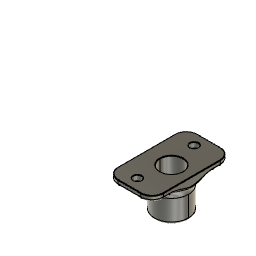
CurtainRodBracket_F3-01_004 (Side Mount) (Autodesk Fusion 360 design; units mm, degrees)
Autodesk Fusion 360 part; units mm, degrees
box "BoxPrimitive1" add length 70 width 30 height 5 placed x (0, 1, 0) y (-1, 0, 0) z (0, 0, 1) at (30, -5, 0) makes body 1
box "BoxPrimitive2" add length 30 width 30 height 25 placed x (0, 1, 0) y (-1, 0, 0) z (0, 0, 1) at (30, 15, 5) bodies 1
cylinder "CylinderPrimitive1" cut diameter 20 height -40 placed x (0, 0, -1) y (0, 1, 0) z (1, 0, 0) at (30, 30, 15) bodies 1
fillet "Fillet1" radius 14 2 edges at (15, 15, 30) (15, 45, 30) on bodies 1
fillet "Fillet2" radius 10 2 edges at (15, 15, 5) (15, 45, 5) on bodies 1
box "BoxPrimitive4" add length 20 width 30 height 7 placed x (0, 1, 0) y (1, 0, 0) z (0, 0, -1) at (0, -5, 0) bodies 1
cylinder "CylinderPrimitive3" cut diameter 7 height 21 placed x (1, 0, 0) y (0, 1, 0) z (0, 0, 1) at (15, 5, 0) bodies 1
cylinder "CylinderPrimitive4" cut diameter 20 height 34 placed x (1, 0, 0) y (0, 1, 0) z (0, 0, 1) at (15, 5, 5) bodies 1
fillet "Fillet3" radius 1.4 1 edges at (15, 15, 5) on bodies 1
fillet "Fillet4" radius 5 4 edges at (5.8399, 7.6914, 5.3692) (10.0517, 13.6899, 10.0517) (19.9483, 13.6899, 10.0517) (24.1593, 7.6637, 5.3615) on bodies 1
ref_plane "WorkPlane1" through (15, 30, 2.5) normal (0, -1, 0) x (0, 0, 1)
fillet "Fillet5" radius 10 2 edges at (30, -5, -1) (0, -5, -1) on bodies 1
fillet "Fillet6" radius 2 19 edges at (30, 60, 5) (30, 47.9289, 7.9289) (30, 45, 15.5) (30, 40.8995, 25.8995) (30, 30, 30) (30, 19.1005, 25.8995) (30, 15, 15.5) (30, 12.0711, 7.9289) (27.0711, -2.0711, 5) (15, -5, 5) (2.9289, -2.0711, 5) (0, 12.0711, 7.9289) (0, 15, 15.5) (0, 19.1005, 25.8995) (0, 30, 30) (0, 40.8995, 25.8995) (0, 45, 15.5) (0, 47.9289, 7.9289) (0, 60, 5) on bodies 1
fillet "Fillet7" radius 1 2 edges at (30, 20.6767, 18.6162) (0, 20.6767, 11.3838) on bodies 1
box "BoxPrimitive3" cut length 65 width 106 height -57 placed x (0, 0, -1) y (1, 0, 0) z (0, -1, 0) at (-44, 30, 51.5) bodies 1
fillet "Fillet9" radius 10 2 edges at (0, 15, -3.5) (30, 15, -3.5) on bodies 1
chamfer "Chamfer2" distance 0.4 angle 45 4 edges at (15, -5, -7) (30, 5, -7) (15, 15, -7) (0, 5, -7) measured on face at (6.666, 5, -7) measured on face at (30, 14.9957, 1.3615) measured on face at (6.666, 5, -7) measured on face at (0, 14.9957, 1.3615) on bodies 1
fillet "Fillet10" radius 2 3 edges at (2.9289, 12.0711, 0) (15, 15, 0) (27.0711, 12.0711, 0) on bodies 1
fillet "Fillet11" radius 3 4 edges at (0, 8.2445, -0.662) (0, 20.8166, 0) (30, 20.8166, 0) (30, 8.2445, -0.662) on bodies 1
cylinder "CylinderPrimitive5" cut diameter 7 height -50 placed x (1, 0, 0) y (0, 1, 0) z (0, 0, 1) at (15, 5, 5) bodies 1
chamfer "Chamfer3" distance 0.4 angle 45 2 edges at (11.7369, 6.2657, 5) (16.2657, 1.7369, -7) measured on face at (14.8594, -1.4915, 5) measured on face at (14.8594, 12.5582, -7) on bodies 1
box "BoxPrimitive5" add length 1 width 2 height 0.5 placed x (0, -1, 0) y (-1, 0, 0) z (0, 0, -1) at (20, -3.5, -7) separate body makes body 2
chamfer "Chamfer4" distance 0.5 angle 45 4 edges at (20, -4, -7.5) (19, -4.5, -7.5) (19, -3.5, -7.5) (18, -4, -7.5) measured on face at (18.6667, -3.8333, -7.5) measured on face at (18.6667, -3.8333, -7.5) measured on face at (18.6667, -3.8333, -7.5) measured on face at (18.6667, -3.8333, -7.5) on bodies 2
copy_body "CopyPasteBodies1" bodies 2 makes body 3
move_body "Move1" bodies 3 to x (1, 0, 0) y (0, 1, 0) z (0, 0, 1) at (9, 9, 0)
copy_body "CopyPasteBodies2" bodies 2 makes body 4
move_body "Move2" bodies 4 to x (1, 0, 0) y (0, 1, 0) z (0, 0, 1) at (-17, 9, 0)
move_body "Move3" bodies 2 to x (0, -1, 0) y (1, 0, 0) z (0, 0, 1) at (23.5, 15.5, 0)
copy_body "CopyPasteBodies3" bodies 2 makes body 5
move_body "Move4" bodies 5 to x (1, 0, 0) y (0, 1, 0) z (0, 0, 1) at (-9, 0, 0)
copy_body "CopyPasteBodies4" bodies 2 5 makes body 6 makes body 7
move_body "Move5" bodies 6 7 to x (1, 0, 0) y (0, 1, 0) z (0, 0, 1) at (0, 17, 0)
copy_body "CopyPasteBodies5" bodies 7 makes body 8
move_body "Move6" bodies 8 to x (1, 0, 0) y (0, 1, 0) z (0, 0, 1) at (25, 0, 0)
combine "Combine1" operation add target body 1 tool bodies 2 3 4 5 6 7
mirror "Mirror1" about plane through (15, 30, 2.5) normal (0, -1, 0) of bodies 1 merged
ref_plane "WorkPlane2" through (75, 30, 13) normal (1, 0, 0) x (0, 0, -1)
box "BoxPrimitive6" add length 40 width 70 height 5 placed x (0, 0, 1) y (0, -1, 0) z (1, 0, 0) at (75, 65, -7) separate body makes body 9
cylinder "CylinderPrimitive6" add diameter 30 height 30 placed x (0, 0, -1) y (0, 1, 0) z (1, 0, 0) at (80, 30, 15) bodies 9
cylinder "CylinderPrimitive7" cut diameter 20 height -47 placed x (0, 0, -1) y (0, 1, 0) z (1, 0, 0) at (110, 30, 15) bodies 9
fillet "Fillet12" radius 10 1 edges at (80, 35.4242, 28.9849) on bodies 9
fillet "Fillet13" radius 2 1 edges at (110, 24.5758, 28.9849) on bodies 9
fillet "Fillet14" radius 1 1 edges at (110, 20.6767, 18.6162) on bodies 9
fillet "Fillet15" radius 10 4 edges at (77.5, -5, 33) (77.5, -5, -7) (77.5, 65, 33) (77.5, 65, -7) on bodies 9
cylinder "CylinderPrimitive8" cut diameter 7 height -15 placed x (0, 0, -1) y (0, 1, 0) z (1, 0, 0) at (80, 5, 10) bodies 9
cylinder "CylinderPrimitive9" cut diameter 20 height 24 placed x (0, 0, -1) y (0, 1, 0) z (1, 0, 0) at (80, 5, 10) bodies 9
fillet "Fillet16" radius 1.4 1 edges at (80, 14.8058, 11.9612) on bodies 9
fillet "Fillet17" radius 4 3 edges at (80.3437, 7.9669, 19.0446) (86.7888, 14.6582, 12.5923) (80.3437, 11.2174, 2.7922) on bodies 9
fillet "Fillet18" radius 2 14 edges at (82.8586, 30, 33) (82.8586, 30, 33) (80, 51.1747, 33) (80, 8.8253, 33) (80, 62.0711, 30.0711) (80, 65, 13) (80, 62.0711, -4.0711) (80, 48.4372, -7) (80.4606, 30, -7) (80, 11.5628, -7) (80, -2.0711, -4.0711) (80, -5, 13) (80, -2.0711, 30.0711) (80, 8.8253, 33) on bodies 9
chamfer "Chamfer5" distance 0.4 angle 45 8 edges at (75, -5, 13) (75, -2.0711, -4.0711) (75, 30, -7) (75, 62.0711, -4.0711) (75, 65, 13) (75, 62.0711, 30.0711) (75, 30, 33) (75, -2.0711, 30.0711) measured on face at (75, 56.6573, 13.4176) measured on face at (76, -4.9547, 2.0494) measured on face at (75, 56.6573, 13.4176) measured on face at (76, 64.9887, 2.5242) measured on face at (75, 56.6573, 13.4176) measured on face at (76, 55.4758, 32.9887) measured on face at (75, 56.6573, 13.4176) measured on face at (76, 4.0494, 32.9547) on bodies 9
chamfer "Chamfer6" distance 0.4 angle 45 2 edges at (75, 20.6767, 11.3838) (75, 1.7369, 8.7343) measured on face at (75, 56.3907, 13.4176) measured on face at (75, 56.3907, 13.4176) on bodies 9
chamfer "Chamfer7" distance 0.4 angle 45 1 edges at (80, 1.7369, 8.7343) measured on face at (76.9333, 4.8255, 6.5044) on bodies 9
box "BoxPrimitive7" cut length 79.8249 width 114.6289 height -125 placed x (0, 0, -1) y (1, 0, 0) z (0, -1, 0) at (47.2286, 30, 46.964) bodies 9
move_body "Move8" bodies 8 to x (0, 0, -1) y (0, 1, 0) z (1, 0, 0) at (82, -17, 45.5)
copy_body "CopyPasteBodies6" bodies 8 makes body 10
move_body "Move9" bodies 10 to x (1, 0, 0) y (0, 1, 0) z (0, 0, 1) at (0, 22, 5)
copy_body "CopyPasteBodies7" bodies 8 makes body 11
move_body "Move10" bodies 11 to x (1, 0, 0) y (0, 0, 1) z (0, -1, 0) at (0, 15, -1)
copy_body "CopyPasteBodies8" bodies 11 makes body 12
move_body "Move11" bodies 12 to x (1, 0, 0) y (0, 1, 0) z (0, 0, 1) at (0, 0, 35)
copy_body "CopyPasteBodies9" bodies 8 makes body 13
move_body "Move12" bodies 13 to x (1, 0, 0) y (0, 1, 0) z (0, 0, 1) at (0, 0, 11)
move_body "Move13" bodies 8 to x (1, 0, 0) y (0, 1, 0) z (0, 0, 1) at (0, 0, -5)
combine "Combine2" operation add target body 13 tool bodies 12 11 10 9 8
mirror "Mirror2" about plane through (15, 30, 2.5) normal (0, -1, 0) of bodies 13 merged
sketch "Sketch23" plane through (80, 0, 0) normal (1, 0, 0) x (0, 1, 0)
  line L0 (45, -5) -> (55, -5)
  arc A0 (55, -5) -> (63, 3) centre (55, 3) ccw
  line L1 (63, 3) -> (63, 23)
  arc A1 (63, 23) -> (55, 31) centre (55, 23) ccw
  line L2 (55, 31) -> (49.2094, 31)
  arc A2 (54.74, 18.5961) -> (49.2094, 31) centre (30, 15) ccw
  arc A3 (54.74, 18.5961) -> (51.4538, 2.1652) centre (55, 10) ccw
  arc A4 (45, -5) -> (51.4538, 2.1652) centre (30, 15) ccw
  circle A5 centre (55, 10) radius 3.9
  line L3 (61, 7.6363) -> (49.7386, 7.6363) construction
  line L4 (49.7386, 7.6363) -> (49.7386, -2) construction
  line L5 (49.7386, -2) -> (61, -2) construction
  line L6 (61, -2) -> (61, 7.6363) construction
  text T0 "Up" font "Arial" height 5 align left top in box 11.2614 x 9.6363 at (61, 7.6363) x (-1, 0) y (0, -1) spacing 1 kerned
extrude "Extrude2" cut sketch "Sketch23" against normal blind 0.5 text T0 bodies 13
move_body "Move7" bodies 13 to x (0, 0, -1) y (0, 1, 0) z (1, 0, 0) at (76.5, 0, 27.5)
box "BoxPrimitive8" cut length 91 width 55 height 6 placed x (0, -1, 0) y (1, 0, 0) z (0, 0, 1) at (62, 75, -47.5) bodies 13
hidden bodies 1
